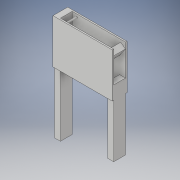
# Autodesk Inventor part: PBotCatapultShell
Saved by Autodesk Inventor 2018 (Build 220112000, 112)
## iProperties
Created: 2018-05-31
Part Number: PBotCatapultShell
Material: Generic
Document SubType Name: Modeling
Designer: choices
Density: 1 g/cm^3
Appearance: Default
Author: choices
Autodesk Inventor part; units mm, degrees
ref_plane "YZ Plane" through (0, 0, 0) normal (1, 0, 0) x (0, 1, 0)
ref_plane "XZ Plane" through (0, 0, 0) normal (0, 1, 0) x (-1, 0, 0)
ref_plane "XY Plane" through (0, 0, 0) normal (0, 0, 1) x (1, 0, 0)
sketch "Sketch1" plane through (0, 0, 0) normal (0, 1, 0) x (-1, 0, 0)
  line L0 (0, 0) -> (50.8, 0)
  line L1 (50.8, 0) -> (50.8, -101.6)
  line L2 (50.8, -101.6) -> (0, -101.6)
  line L3 (0, -101.6) -> (0, 0)
  dimension "d0" = 50.8
  dimension "d1" = 101.6
  constraints: 8 end point, 2 parallel, 1 horizontal, 1 perpendicular
  measures "d0" distance of L1.end L2.end
  measures "d1" distance of L0.end L1.end
extrude "Extrusion1" add sketch "Sketch1" along normal blind 914.4
sketch "Sketch2" plane through (-50.8, 0, 0) normal (0, 0, 1) x (1, 0, 0)
  line L0 (0, 0) -> (0, 914.4) projected
  line L1 (0, 914.4) -> (508, 914.4)
  line L2 (508, 914.4) -> (508, 533.4)
  line L3 (508, 533.4) -> (0, 533.4)
  line L4 (0, 533.4) -> (0, 914.4)
  point P0 (50.8, 0)
  dimension "d4" = 508
  dimension "d5" = 381
  constraints: 8 end point, 2 parallel, 1 horizontal, 1 perpendicular
  measures "d4" distance of L2.end L3.end
  measures "d5" distance of L1.end L2.end
extrude "Extrusion2" add sketch "Sketch2" along normal blind 12.7
sketch "Sketch3" plane through (0, 0, -101.6) normal (0, 0, -1) x (-1, 0, 0)
  line L0 (0, 533.4) -> (0, 914.4) projected
  line L1 (0, 914.4) -> (-457.2, 914.4) projected
  line L2 (-457.2, 914.4) -> (-457.2, 533.4) projected
  line L3 (-457.2, 533.4) -> (0, 533.4) projected
  line L4 (-457.2, 914.4) -> (50.8, 914.4) projected
  line L5 (50.8, 914.4) -> (50.8, 533.4) projected
  line L6 (50.8, 533.4) -> (-457.2, 533.4) projected
  line L7 (-457.2, 533.4) -> (-457.2, 914.4) projected
  point P0 (0, 0)
extrude "Extrusion3" add sketch "Sketch3" along normal blind 12.7
sketch "Sketch4" plane through (0, 0, -101.6) normal (0, 0, 1) x (1, 0, 0)
  line L0 (457.2, 533.4) -> (0, 533.4) projected
  line L1 (457.2, 533.4) -> (406.4, 533.4)
  line L2 (406.4, 533.4) -> (406.4, 647.7)
  line L3 (406.4, 647.7) -> (457.2, 647.7)
  line L4 (457.2, 647.7) -> (457.2, 533.4)
  line L5 (406.4, 647.7) -> (457.2, 647.7)
  line L6 (457.2, 647.7) -> (457.2, 76.2)
  line L7 (457.2, 76.2) -> (406.4, 76.2)
  line L8 (406.4, 76.2) -> (406.4, 647.7)
  line L9 (457.2, 914.4) -> (-50.8, 914.4) projected
  point P0 (0, 0)
  dimension "d10" = 50.8
  dimension "d11" = 114.3
  dimension "d12" = 838.2
  constraints: 16 end point, 4 parallel, 2 horizontal, 2 perpendicular, 1 point on line
  measures "d10" distance of L2.end L3.end
  measures "d11" distance of L1.end L2.end
  measures "d12" distance between parallel lines of L7 L9
extrude "Extrusion4" add sketch "Sketch4" along normal up to surface (101.6 mm away)
sketch "Sketch5" plane through (0, 0, -101.6) normal (0, 0, 1) x (1, 0, 0)
  circle A0 centre (38.1, 889) radius 6.35
  circle A1 centre (292.1, 647.7) radius 6.35
  line L0 (-50.8, 914.4) -> (-50.8, 533.4) projected
  line L1 (457.2, 914.4) -> (-50.8, 914.4) projected
  line L2 (457.2, 533.4) -> (457.2, 914.4) projected
  line L3 (-50.8, 533.4) -> (457.2, 533.4) projected
  point P0 (0, 0)
  dimension "d15" = 12.7
  dimension "d16" = 12.7
  dimension "d17" = 88.9
  dimension "d18" = 25.4
  dimension "d20" = 165.1
  dimension "d21" = 114.3
  constraints: 2 centre point
  measures "d15" diameter of A0
  measures "d16" diameter of A1
  measures "d17" distance from line of L0 A0.centre
  measures "d18" distance from line of L1 A0.centre
  measures "d20" distance from line of L2 A1.centre
  measures "d21" distance from line of L3 A1.centre
extrude "Extrusion5" add sketch "Sketch5" along normal up to surface (101.6 mm away) contours A0 | A1
sketch "Sketch6" plane through (0, 0, -101.6) normal (0, 0, 1) x (1, 0, 0)
  line L0 (457.2, 914.4) -> (457.2, 647.7) projected
  line L1 (457.2, 863.6) -> (406.2091, 790.7774)
  line L2 (457.2, 863.6) -> (546.1, 863.6) construction
  line L3 (406.2091, 790.7774) -> (364.5961, 819.9151)
  line L4 (364.5961, 819.9151) -> (415.5871, 892.7377)
  line L5 (415.5871, 892.7377) -> (457.2, 863.6)
  line L6 (457.2, 914.4) -> (0, 914.4) projected
  point P0 (0, 0)
  dimension "d24" = 88.9
  dimension "d25" = 125
  dimension "d26" = 50.8
  dimension "d27" = 50.8
  constraints: 10 end point, 3 perpendicular, 1 equal length, 1 horizontal, 1 point on line
  measures "d24" distance of L1.start L1.end
  measures "d25" angle of L1 L2
  measures "d26" distance of L1.end L3.end
  measures "d27" distance from line of L6 L1.start
extrude "Extrusion6" add sketch "Sketch6" along normal up to surface (101.6 mm away)
body "Solid1"
